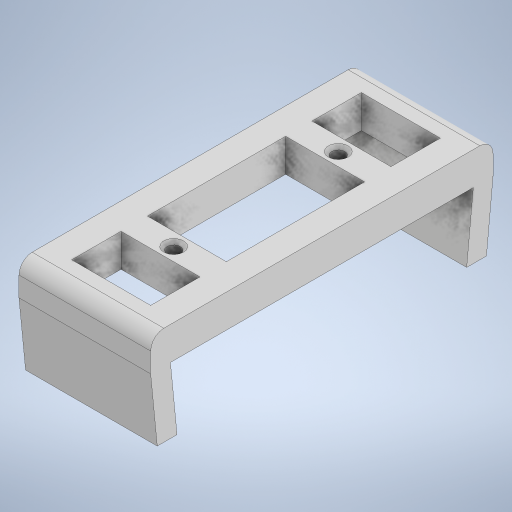
# Autodesk Inventor part: 스텝모터 상판
Saved by Autodesk Inventor 2023 (Build 270158000, 158)
## iProperties
Created: 2022-11-11
Part Number: 스텝모터 상판
Material: 일반
Document SubType Name: Modeling
Designer: hyunsu
Density: 1 g/cm^3
Appearance: 기본값
Author: hyunsu
Autodesk Inventor part; units mm, degrees
ref_plane "YZ Plane" through (0, 0, 0) normal (1, 0, 0) x (0, 1, 0)
ref_plane "XZ Plane" through (0, 0, 0) normal (0, 1, 0) x (-1, 0, 0)
ref_plane "XY Plane" through (0, 0, 0) normal (0, 0, 1) x (1, 0, 0)
sketch "스케치1" plane through (0, 0, 0) normal (0, 1, 0) x (-1, 0, 0)
  line L0 (10, 26) -> (-10, 26)
  line L1 (-10, 26) -> (-10, -26)
  line L2 (-10, -26) -> (10, -26)
  line L3 (10, -26) -> (10, 26)
  line L4 (10, 26) -> (-10, -26) construction
  line L5 (-10, 26) -> (10, -26) construction
  line L6 (6, 22) -> (-6, 22)
  line L7 (-6, 22) -> (-6, -22)
  line L8 (-6, -22) -> (6, -22)
  line L9 (6, -22) -> (6, 22)
  line L10 (7.75, 10.5) -> (-7.75, 10.5)
  line L11 (-7.75, 10.5) -> (-7.75, -10.5) construction
  line L12 (-7.75, -10.5) -> (7.75, -10.5)
  line L13 (7.75, -10.5) -> (7.75, 10.5) construction
  line L14 (7.75, 10.5) -> (-7.75, -10.5) construction
  line L15 (-7.75, 10.5) -> (7.75, -10.5) construction
  line L16 (6, 14.5) -> (-6, 14.5)
  line L17 (0, 0) -> (3.5234, 0)
  line L18 (6, -14.5) -> (-6, -14.5)
  point P0 (0, 10.5)
  point P1 (-6, 10.5)
  point P2 (6, 10.5)
  point P3 (6, -10.5)
  point P4 (-6, -10.5)
  dimension "d0" = 20
  dimension "d1" = 52
  dimension "d2" = 4
  dimension "d3" = 15.5
  dimension "d4" = 21
  dimension "d5" = 4
  constraints: 38 end point, 6 parallel, 5 midpoint, 4 perpendicular, 3 horizontal, 2 point on line, 2 symmetric about line, 3 other
  measures "d0" distance of L2.end L1.end
  measures "d1" distance of L1.end L0.end
  measures "d2" distance between parallel lines of L3 L9
  measures "d3" distance of L12.end L11.end
  measures "d4" distance of L11.end L10.end
  measures "d5" distance from line of point (0, 10.5) L16
extrude "돌출1" add sketch "스케치1" along normal blind 5 contours L3 L2 L1 L0 | L9 L10 L7 L16 | L9 L18 L7 L12
sketch "스케치2" plane through (0, 5, 0) normal (0, 1, 0) x (1, 0, 0)
  circle A0 centre (0, -12.5) radius 1
  line L0 (0, 0) -> (-3.3387, 0)
  line L1 (6, -10.5) -> (-6, -10.5) projected
  circle A1 centre (0, 12.5) radius 1
  dimension "d8" = 2
  dimension "d9" = 2
  constraints: 2 centre point, 2 end point, 1 horizontal, 1 symmetric about line, 1 vertical alignment, 1 other
  measures "d8" diameter of A0
  measures "d9" distance from line of L1 A0.centre
hole "구멍1" at (0, 5, 12.5) at (0, 5, -12.5) direction (0, -1, 0) diameter 2 end through all countersink diameter 3 countersink angle 90
sketch "스케치3" plane through (10, 0, 26) normal (1, 0, 0) x (0, 0, -1)
  line L0 (0, 0) -> (1, -10)
  line L1 (1, -10) -> (4, -10)
  line L2 (4, -10) -> (2.9751, 0.2492)
  line L3 (0, 0) -> (52, 0) projected
  line L4 (26, 0) -> (26, -7.8)
  line L5 (52, 0) -> (51, -10)
  line L6 (51, -10) -> (48, -10)
  line L7 (48, -10) -> (49.0249, 0.2492)
  point P0 (49, 0)
  point P1 (3, 0)
  dimension "d17" = 10
  dimension "d18" = 4
  dimension "d19" = 3
  constraints: 14 end point, 3 symmetric about line, 1 horizontal, 1 parallel, 1 vertical, 1 other
  measures "d17" distance of the line from the sketch origin of L1
  measures "d18" horizontal distance of L0.start L1.end
  measures "d19" distance of L0.end L1.end
extrude "돌출2" add sketch "스케치3" against normal up to surface (20 mm away)
fillet "모깎기1" radius 2 2 edges at (0, 5, 26) (0, 5, -26)
